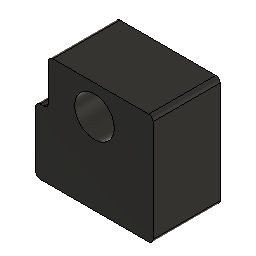
StandoffHolder (Autodesk Fusion 360 design; units mm, degrees)
Autodesk Fusion 360 part; units mm, degrees
sketch "Sketch1" plane through (0, -6.35, 0) normal (0, -1, 0) x (1, 0, 0)
  line L0 (-4.7475, -5.207) -> (-4.7475, 3.8619)
  line L1 (-4.7475, 3.8619) -> (-6.3477, 3.8619)
  line L2 (-6.3477, 3.8619) -> (-6.3477, -5.2324)
  arc A0 (-6.3477, -5.2324) -> (-3.9601, -7.62) centre (-3.9601, -5.2324) ccw
  line L3 (-3.9601, -7.62) -> (16.6647, -7.62)
  arc A1 (16.6647, -7.62) -> (19.0523, -5.2324) centre (16.6647, -5.2324) ccw
  line L4 (19.0523, -5.2324) -> (19.0523, 3.8619)
  line L5 (19.0523, 3.8619) -> (17.4521, 3.8619)
  line L6 (17.4521, 3.8619) -> (17.4521, -5.207)
  arc A2 (16.6393, -6.0198) -> (17.4521, -5.207) centre (16.6393, -5.207) ccw
  line L7 (16.6393, -6.0198) -> (-3.9347, -6.0198)
  arc A3 (-4.7475, -5.207) -> (-3.9347, -6.0198) centre (-3.9347, -5.207) ccw
  line L8 (-3.9199, -6.0198) -> (16.6245, -6.0198)
  line L9 (17.4521, -5.1922) -> (17.4521, 14.1076)
  line L10 (16.6245, 14.9352) -> (-1.528, 14.9352)
  line L11 (-4.7475, 5.5118) -> (-4.7475, -5.1922)
  arc A4 (-4.7475, -5.1922) -> (-3.9199, -6.0198) centre (-3.9199, -5.1922) ccw
  arc A5 (16.6245, -6.0198) -> (17.4521, -5.1922) centre (16.6245, -5.1922) ccw
  arc A6 (17.4521, 14.1076) -> (16.6245, 14.9352) centre (16.6245, 14.1076) ccw
  line L12 (10.0168, 9.3726) -> (0.7463, 9.3726)
  line L13 (6.3523, 14.9352) -> (6.3523, 9.3726)
  circle A7 centre (6.3523, 9.3726) radius 3.7465
  line L14 (-4.7475, 3.8619) -> (-2.3662, 3.8619)
  line L15 (-2.3662, 7.1882) -> (-2.3662, 14.097)
  line L16 (-2.3662, 3.8619) -> (-2.3662, -6.0198)
  line L17 (-3.9093, 6.35) -> (-3.2044, 6.35)
  arc A8 (-1.528, 14.9352) -> (-2.3662, 14.097) centre (-1.528, 14.097) ccw
  arc A9 (-3.9093, 6.35) -> (-4.7475, 5.5118) centre (-3.9093, 5.5118) ccw
  arc A10 (-3.2044, 6.35) -> (-2.3662, 7.1882) centre (-3.2044, 7.1882) ccw
  point P0 (17.4521, -6.0198)
  point P1 (17.4521, 14.9352)
  dimension "d29" = 20.955
  dimension "d30" = 0.8276
  dimension "d31" = 7.493
  dimension "d39" = 2.3813
  dimension "d40" = 0.8382
  dimension "d46" = 5.5626
  constraint perpendicular L6 L8
  constraint perpendicular L8 L9
  constraint perpendicular L9 L10
  constraint perpendicular L8 L11
  constraint tangent L8 A4
  constraint tangent L11 A4
  constraint coincident P0 L8
  constraint coincident P0 L9
  constraint tangent L8 A5
  constraint tangent L9 A5
  constraint equal A4 A5
  constraint coincident P1 L9
  constraint coincident P1 L10
  constraint tangent L9 A6
  constraint tangent L10 A6
  constraint equal A4 A6
  constraint parallel L10 L12
  constraint coincident L12 L13.end
  constraint perpendicular L12 L13
  constraint coincident L13.end A7.centre
  constraint coincident L0.end L1.start
  constraint perpendicular L0 L14
  constraint perpendicular L10 L15
  constraint coincident L8 L16.end
  constraint coincident L7 L16.end
  constraint perpendicular L15 L17
  constraint coincident L10 L13.start
  constraint tangent L15 A8
  constraint tangent L10 A8
  constraint tangent L17 A9
  constraint tangent L11 A9
  constraint equal A8 A9
  constraint coincident L14.end L15
  constraint tangent L17 A10
  constraint tangent L15 A10
  constraint equal A8 A10
  measures "d29" distance of P0 P1
  measures "d30" radius of A4
  measures "d31" diameter of A7
  measures "d39" distance of L0.end L14.end
  measures "d40" radius of A8
  measures "d46" distance of L13.start L13.end
extrude "Extrude1" add sketch "Sketch1" against normal blind 12.7 contours L0 L7 L8 L11 A4 L14 L16 | L6 L7 L8 L9 L10 L11 A5 A6 L14 L15 L16 L17 A8 A9 A10
hole "Hole1" at (12.7, 0, -6.0198) direction (0, 0, 1) diameter 3.429 depth 8.382 tip angle 180
thread "Thread1" "ANSI Unified Screw Threads 0.164(#8) 8-32 UNC 8-32 UNC 2B" major diameter 4.1656 minor diameter 3.4163 pitch 0.7937 angle 60 modelled right hand crest width 0.2341 on face at (12.8707, 1.706, -0.4318) crest through (10.9919, 0, -5.8214)
hole "Hole2" at (0, 0, -6.0198) direction (0, 0, 1) diameter 3.429 depth 8.382 tip angle 180
thread "Thread2" "ANSI Unified Screw Threads 0.164(#8) 8-32 UNC 8-32 UNC 2B" major diameter 4.1656 minor diameter 3.4163 pitch 0.7937 angle 60 modelled right hand crest width 0.2341 on face at (0.1707, 1.706, -0.4318) crest through (-1.7081, 0, -5.8214)
equation "d39 = ( 3 / 32 ) * 1 in"
named bodies: "StandoffHolder"
